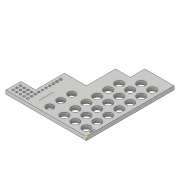
# Autodesk Inventor part: Test laser cutter tolerances
Saved by Autodesk Inventor 2020 (Build 240168000, 168)
## iProperties
Created: 2019-10-14
Part Number: Test laser cutter tolerances
Material: Generic
Document SubType Name: Modeling
Designer: FTC8863
Density: 1 g/cm^3
Appearance: Default
Author: FTC8863
Autodesk Inventor part; units mm, degrees
ref_plane "YZ Plane" through (0, 0, 0) normal (1, 0, 0) x (0, 1, 0)
ref_plane "XZ Plane" through (0, 0, 0) normal (0, 1, 0) x (-1, 0, 0)
ref_plane "XY Plane" through (0, 0, 0) normal (0, 0, 1) x (1, 0, 0)
sketch "Sketch1" plane through (0, 0, 0) normal (0, 1, 0) x (-1, 0, 0)
  line L0 (0, 0) -> (139.7, 0)
  line L1 (139.7, 0) -> (139.7, -152.4)
  line L2 (139.7, -152.4) -> (0, -152.4)
  line L3 (0, -152.4) -> (0, 0)
  line L4 (139.7, -152.4) -> (127, -152.4)
  line L5 (114.3, -76.2) -> (114.3, -26.0366)
  line L6 (114.3, -26.0366) -> (139.7, -26.0366)
  line L7 (139.7, -26.0366) -> (139.7, -152.4)
  line L8 (127, -152.4) -> (76.2, -152.4)
  line L9 (76.2, -127) -> (76.2, -76.2)
  line L10 (76.2, -76.2) -> (114.3, -76.2)
  line L11 (76.2, -152.4) -> (50.8, -152.4)
  line L12 (50.8, -152.4) -> (50.8, -127)
  line L13 (50.8, -127) -> (76.2, -127)
  circle A0 centre (12.7, -12.7) radius 6.35 construction
  circle A1 centre (12.7, -31.75) radius 6.35 construction
  circle A2 centre (12.7, -50.8) radius 6.35 construction
  circle A3 centre (12.7, -69.85) radius 6.35 construction
  circle A4 centre (12.7, -88.9) radius 6.35 construction
  circle A5 centre (12.7, -107.95) radius 6.35 construction
  circle A6 centre (12.7, -127) radius 6.35 construction
  circle A7 centre (31.75, -12.7) radius 6.35 construction
  circle A8 centre (31.75, -31.75) radius 6.35 construction
  circle A9 centre (31.75, -50.8) radius 6.35 construction
  circle A10 centre (31.75, -69.85) radius 6.35 construction
  circle A11 centre (31.75, -88.9) radius 6.35 construction
  circle A12 centre (31.75, -107.95) radius 6.35 construction
  circle A13 centre (31.75, -127) radius 6.35 construction
  circle A14 centre (12.7, -12.7) radius 6.873
  circle A15 centre (12.7, -31.75) radius 6.8857
  circle A16 centre (12.7, -50.8) radius 6.8984
  circle A17 centre (12.7, -69.85) radius 6.9111
  circle A18 centre (12.7, -88.9) radius 6.9238
  circle A19 centre (12.7, -107.95) radius 6.9365
  circle A20 centre (12.7, -127) radius 6.9492
  circle A21 centre (31.75, -12.7) radius 6.9619
  circle A22 centre (31.75, -31.75) radius 6.9746
  circle A23 centre (31.75, -50.8) radius 6.9873
  circle A24 centre (31.75, -69.85) radius 7
  circle A25 centre (31.75, -88.9) radius 7.0127
  circle A26 centre (31.75, -107.95) radius 7.0254
  circle A27 centre (31.75, -127) radius 7.0381
  circle A28 centre (50.8, -12.7) radius 7.0635
  circle A29 centre (50.8, -31.75) radius 7.0635
  circle A30 centre (50.8, -50.8) radius 7.0762
  circle A31 centre (50.8, -69.85) radius 7.0889
  circle A32 centre (50.8, -88.9) radius 7.1016
  circle A33 centre (50.8, -107.95) radius 7.0045
  circle A34 centre (76.2, -12.7) radius 6.35
  circle A35 centre (76.2, -31.75) radius 6.35
  circle A36 centre (76.2, -50.8) radius 6.35
  line L14 (6.4177, -6.5588) -> (6.4177, -14.6901) construction
  line L15 (8.0052, -4.9713) -> (8.0052, -13.1026) construction
  circle A37 centre (133.35, -6.35) radius 1.778
  circle A38 centre (133.35, -12.7) radius 1.7907
  circle A39 centre (133.35, -19.05) radius 1.8034
  circle A40 centre (127, -6.35) radius 1.8161
  circle A41 centre (127, -12.7) radius 1.8288
  circle A42 centre (127, -19.05) radius 1.8415
  circle A43 centre (120.65, -6.35) radius 1.8542
  circle A44 centre (120.65, -12.7) radius 1.8669
  circle A45 centre (120.65, -19.05) radius 1.8796
  circle A46 centre (114.3, -6.35) radius 1.8923
  circle A47 centre (114.3, -12.7) radius 1.8669
  circle A48 centre (114.3, -19.05) radius 1.8796
  circle A49 centre (107.95, -6.35) radius 1.8923
  circle A50 centre (107.95, -12.7) radius 1.8669
  circle A51 centre (107.95, -19.05) radius 1.8796
  circle A52 centre (107.95, -25.4) radius 1.8923
  circle A53 centre (107.95, -31.75) radius 1.65
  circle A54 centre (107.95, -38.1) radius 1.7
  circle A55 centre (107.95, -44.45) radius 1.75
  circle A56 centre (107.95, -50.8) radius 2.15
  circle A57 centre (107.95, -57.15) radius 2.2
  circle A58 centre (107.95, -63.5) radius 2.25
  dimension "d0" = 139.7
  dimension "d1" = 152.4
  dimension "d3" = 127
  dimension "d5" = 76.2
  dimension "d7" = 25.4
  dimension "d8" = 12.7
  dimension "d9" = 12.7
  dimension "d10" = 12.7
  dimension "d13" = 19.05
  dimension "d16" = 19.05
  dimension "d19" = 13.746
  dimension "d20" = 13.7714
  dimension "d21" = 13.7968
  dimension "d22" = 13.8222
  dimension "d23" = 13.8476
  dimension "d24" = 13.873
  dimension "d25" = 13.8984
  dimension "d26" = 13.9238
  dimension "d27" = 13.9492
  dimension "d28" = 13.9746
  dimension "d29" = 14
  dimension "d30" = 14.0254
  dimension "d31" = 14.0508
  dimension "d32" = 14.0762
  dimension "d33" = 14.127
  dimension "d34" = 14.127
  dimension "d35" = 14.1524
  dimension "d36" = 14.1778
  dimension "d37" = 14.2032
  dimension "d38" = 14.009
  dimension "d39" = 12.7
  dimension "d40" = 12.7
  dimension "d41" = 12.7
  dimension "d44" = 50.8
  dimension "d45" = 25.4
  dimension "d46" = 25.4
  dimension "d47" = 3.556
  dimension "d48" = 6.35
  dimension "d49" = 6.35
  dimension "d50" = 3.5814
  dimension "d51" = 6.35
  dimension "d52" = 3.6068
  dimension "d53" = 6.35
  dimension "d54" = 3.6322
  dimension "d55" = 6.35
  dimension "d56" = 3.6576
  dimension "d57" = 3.683
  dimension "d58" = 3.7084
  dimension "d59" = 6.35
  dimension "d60" = 3.7338
  dimension "d61" = 3.7592
  dimension "d62" = 3.7846
  dimension "d63" = 6.35
  dimension "d64" = 3.7338
  dimension "d65" = 3.7592
  dimension "d66" = 3.7846
  dimension "d67" = 6.35
  dimension "d68" = 3.7338
  dimension "d69" = 3.7592
  dimension "d70" = 3.7846
  dimension "d71" = 6.35
  dimension "d72" = 3.3
  dimension "d73" = 3.4
  dimension "d74" = 3.5
  constraints: 59 centre point, 28 end point, 14 coincident, 6 parallel, 5 horizontal, 4 perpendicular, 1 vertical, 26 other
  measures "d0" distance of L1.end L2.end
  measures "d1" distance of L0.end L1.end
  measures "d3" distance of L4.end L5.end
  measures "d5" distance of L8.end L9.end
  measures "d7" distance of L11.end L12.end
  measures "d8" diameter of A0
  measures "d9" distance from line of L0 A0.centre
  measures "d10" distance from line of L3 A0.centre
  measures "d13" distance of A0.centre A1.centre
  measures "d16" distance of A0.centre A7.centre
  measures "d19" diameter of A14
  measures "d20" diameter of A15
  measures "d21" diameter of A16
  measures "d22" diameter of A17
  measures "d23" diameter of A18
  measures "d24" diameter of A19
  measures "d25" diameter of A20
  measures "d26" diameter of A21
  measures "d27" diameter of A22
  measures "d28" diameter of A23
  measures "d29" diameter of A24
  measures "d30" diameter of A25
  measures "d31" diameter of A26
  measures "d32" diameter of A27
  measures "d33" diameter of A28
  measures "d34" diameter of A29
  measures "d35" diameter of A30
  measures "d36" diameter of A31
  measures "d37" diameter of A32
  measures "d38" diameter of A33
  measures "d39" diameter of A34
  measures "d40" diameter of A35
  measures "d41" diameter of A36
  measures "d44" distance between parallel lines of L3 L12
  measures "d45" distance between parallel lines of L12 L9
  measures "d46" distance between parallel lines of L7 L5
  measures "d47" diameter of A37
  measures "d48" distance from line of A37.centre L1
  measures "d49" distance from line of A37.centre L0
  measures "d50" diameter of A38
  measures "d51" distance of A38.centre A37.centre
  measures "d52" diameter of A39
  measures "d53" distance of A39.centre A38.centre
  measures "d54" diameter of A40
  measures "d55" distance of A40.centre A37.centre
  measures "d56" diameter of A41
  measures "d57" diameter of A42
  measures "d58" diameter of A43
  measures "d59" distance of A43.centre A40.centre
  measures "d60" diameter of A44
  measures "d61" diameter of A45
  measures "d62" diameter of A46
  measures "d63" distance of A46.centre A43.centre
  measures "d64" diameter of A47
  measures "d65" diameter of A48
  measures "d66" diameter of A49
  measures "d67" distance of A49.centre A46.centre
  measures "d68" diameter of A50
  measures "d69" diameter of A51
  measures "d70" diameter of A52
  measures "d71" vertical distance of A52.centre A39.centre
  measures "d72" diameter of A53
  measures "d73" diameter of A54
  measures "d74" diameter of A55
extrude "Extrusion1" add sketch "Sketch1" along normal blind 6.35 contours L0 L1 L6 L5 L10 L9 L13 L12 L2 L3
sketch "Sketch2" plane through (0, 6.35, 0) normal (0, 1, 0) x (1, 0, 0)
  line L0 (-4.5975, 9.3875) -> (-4.5975, 17.5188) construction
  line L1 (-4.5975, 17.5188) -> (-1.4235, 17.5188) construction
  line L2 (-1.4235, 17.5188) -> (-1.4235, 9.3875) construction
  line L3 (-1.4235, 9.3875) -> (-4.5975, 9.3875) construction
  point P0 (0, 0)
  constraints: 2 other
sketch "Sketch3" plane through (0, 6.35, 0) normal (0, 1, 0) x (1, 0, 0)
  point P0 (0, 0)
sketch "Sketch4" plane through (0, 6.35, 0) normal (0, 1, 0) x (1, 0, 0)
  line L0 (-95.25, 12.7) -> (-95.2246, 12.7)
  line L1 (-95.2246, 12.7) -> (-95.2246, 38.1)
  line L2 (-95.2246, 38.1) -> (-95.25, 38.1)
  line L3 (-95.25, 38.1) -> (-95.25, 12.7)
  line L4 (-139.7, 26.0366) -> (-139.7, 0) projected
  line L5 (-139.7, 0) -> (0, 0) projected
  dimension "d84" = 0.0254
  dimension "d85" = 25.4
  dimension "d86" = 44.45
  dimension "d87" = 12.7
  constraints: 8 end point, 2 parallel, 1 horizontal, 1 perpendicular
  measures "d84" distance of L2.end L1.end
  measures "d85" distance of L1.end L0.end
  measures "d86" distance between parallel lines of L4 L3
  measures "d87" distance from line of L5 L0.end
extrude "Extrusion2" cut sketch "Sketch4" against normal through all
body "Solid1"
